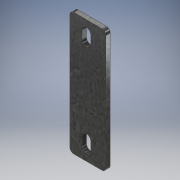
# Autodesk Inventor part: CAR LATERAL BEARING HOLDER
Saved by Autodesk Inventor 2017 (Build 210142000, 142)
## iProperties
Part Number: CAR LATERAL BEARING HOLDER
Material: Genérico
Document SubType Name: Modeling
Designer: Cristian
Density: 1 g/cm^3
Appearance: Valor por defecto
Author: Cristian
Autodesk Inventor part; units mm, degrees
ref_plane "YZ Plane" through (0, 0, 0) normal (1, 0, 0) x (0, 1, 0)
ref_plane "XZ Plane" through (0, 0, 0) normal (0, 1, 0) x (-1, 0, 0)
ref_plane "XY Plane" through (0, 0, 0) normal (0, 0, 1) x (1, 0, 0)
sketch "Boceto1" plane through (0, 0, 0) normal (0, 1, 0) x (-1, 0, 0)
  line L0 (41.275, 139.7) -> (0, 139.7)
  line L1 (0, 139.7) -> (0, 0)
  line L2 (0, 0) -> (41.275, 0)
  line L3 (41.275, 0) -> (41.275, 139.7)
  dimension "d0" = 139.7
  dimension "d1" = 41.275
  constraints: 8 end point, 2 parallel, 1 horizontal, 1 perpendicular
  measures "d0" distance of L2.end L0.start
  measures "d1" distance of L0.start L0.end
extrude "Extrusión1" add sketch "Boceto1" along normal blind 5
sketch "Boceto2" plane through (0, 5, 0) normal (0, 1, 0) x (1, 0, 0)
  circle A0 centre (-22.225, -122.2375) radius 5
  line L0 (-41.275, -139.7) -> (0, -139.7) projected
  circle A1 centre (-22.225, -126.9609) radius 5
  circle A2 centre (-22.225, -117.5141) radius 5
  line L1 (-22.225, -126.9609) -> (-22.225, -122.2375)
  line L2 (-22.225, -122.2375) -> (-22.225, -117.5141)
  line L3 (-41.275, -139.7) -> (-41.275, 0) projected
  line L4 (-17.225, -126.9609) -> (-17.225, -117.5141)
  line L5 (-27.225, -126.9609) -> (-27.225, -117.5141)
  circle A3 centre (-22.225, -17.4625) radius 5
  circle A4 centre (-22.225, -22.1859) radius 5
  circle A5 centre (-22.225, -12.7391) radius 5
  line L6 (-22.225, -22.1859) -> (-22.225, -17.4625)
  line L7 (-22.225, -17.4625) -> (-22.225, -12.7391)
  line L8 (0, 0) -> (-41.275, 0) projected
  line L9 (-27.225, -22.1859) -> (-27.225, -12.7391)
  line L10 (-17.225, -22.1859) -> (-17.225, -12.7391)
  dimension "d4" = 10
  dimension "d5" = 17.4625
  dimension "d6" = 10
  dimension "d7" = 10
  dimension "d8" = 19.4469
  dimension "d9" = 19.05
  dimension "d10" = 10
  dimension "d11" = 10
  dimension "d12" = 10
  dimension "d13" = 19.4469
  dimension "d14" = 19.05
  dimension "d15" = 17.4625
  constraints: 16 end point, 8 point on circle, 7 tangent, 6 centre point, 4 collinear, 3 vertical
  measures "d4" diameter of A0
  measures "d5" distance from line of L0 L1.end
  measures "d6" diameter of A1
  measures "d7" diameter of A2
  measures "d9" distance from line of L3 L1.end
  measures "d10" diameter of A3
  measures "d11" diameter of A4
  measures "d12" diameter of A5
  measures "d14" distance from line of L3 L6.end
  measures "d15" distance from line of L8 L6.end
extrude "Extrusión2" cut sketch "Boceto2" against normal up to next
fillet "Empalme1" radius 4.7625 4 edges at (0, 2.5, 139.7) (-41.275, 2.5, 139.7) (0, 2.5, 0) (-41.275, 2.5, 0)
